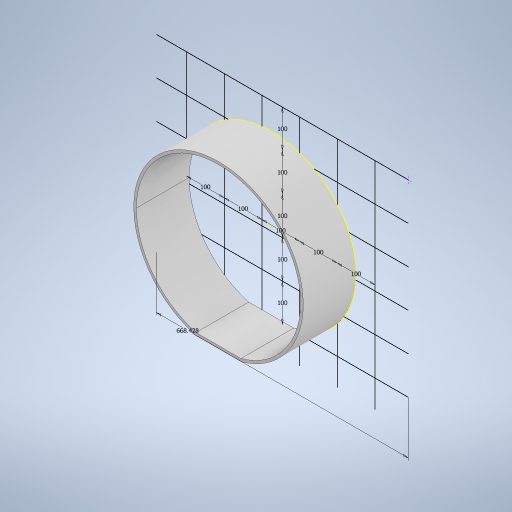
# Autodesk Inventor part: 본체
Saved by Autodesk Inventor 2023 (Build 270158000, 158)
## iProperties
Created: 2022-10-18
Part Number: 본체
Material: 일반
Document SubType Name: Sheet Metal
Designer: ghkdr
Density: 1 g/cm^3
Sheet Metal Rule: 기본값_mm
Appearance: 기본값
Author: ghkdr
Autodesk Inventor part; units mm, degrees
ref_plane "YZ Plane" through (0, 0, 0) normal (1, 0, 0) x (0, 1, 0)
ref_plane "XZ Plane" through (0, 0, 0) normal (0, 1, 0) x (-1, 0, 0)
ref_plane "XY Plane" through (0, 0, 0) normal (0, 0, 1) x (1, 0, 0)
sketch "스케치1" plane through (0, 0, 0) normal (0, 0, 1) x (1, 0, 0)
  line L0 (0.6532, 285.5724) -> (608.6579, 285.5724)
  circle A0 centre (304.6555, 285.5724) radius 26
  spline S0 degree 3 poles (86.6555, 285.5724) (86.6555, 279.2201) (86.9408, 272.7726) (88.3516, 257.3036) (89.7551, 248.2286) (93.8149, 230.0774) (96.4717, 221.0019) (103.0602, 203.1009) (106.9922, 194.2762) (116.0838, 177.1357) (121.2434, 168.8206) (132.6721, 152.9416) (138.9408, 145.3783) (152.4073, 131.206) (159.6045, 124.5975) (174.7019, 112.4806) (182.6013, 106.9724) (198.8544, 97.1353) (207.2073, 92.8062) (224.1185, 85.3392) (232.6761, 82.2009) (242.4395, 79.2689) (243.6563, 78.9149) (244.8727, 78.5724) (284.3294, 78.5724) (323.7861, 78.5724) (363.6413, 78.5724) (364.0398, 78.5724) (364.4384, 78.5724) (370.5905, 80.3047) (376.756, 82.3303) (391.4225, 87.8987) (399.8982, 91.7264) (416.5023, 100.5755) (424.6301, 105.597) (440.2863, 116.7839) (447.814, 122.9492) (462.031, 136.3053) (468.7195, 143.4958) (481.0552, 158.7216) (486.7018, 166.7563) (496.8069, 183.4416) (501.2652, 192.0915) (508.9155, 209.752) (512.1076, 218.7618) (517.2191, 236.884) (519.1388, 245.9959) (521.7638, 264.0837) (522.4696, 273.0593) (522.6361, 282.6064) (522.6452, 283.3458) (522.6528, 284.4297) (522.6543, 284.7752) (522.6554, 285.278) (522.6556, 285.4441) (522.6555, 285.7395) (522.6554, 285.8872) (522.6543, 286.3307) (522.653, 286.6267) (522.647, 287.5152) (522.6404, 288.1086) (522.6125, 289.8917) (522.5833, 291.0845) (522.463, 294.6739) (522.3394, 297.0818) (521.8333, 304.3448) (521.3155, 309.2392) (519.371, 322.7347) (517.5545, 331.408) (512.6658, 348.7558) (509.593, 357.4298) (502.1569, 374.5328) (497.7932, 382.9611) (487.8114, 399.3127) (482.1931, 407.2352) (469.8134, 422.3247) (463.0523, 429.491) (448.5685, 442.8526) (440.8466, 449.0474) (424.6771, 460.3064) (416.2304, 465.3703) (398.8783, 474.2776) (389.9738, 478.1209) (371.9775, 484.5696) (362.8865, 487.1752) (344.7692, 491.1969) (335.7435, 492.6135) (323.7617, 493.7895) (320.6828, 494.0275) (315.1548, 494.3434) (312.6985, 494.4433) (308.7237, 494.5412) (307.196, 494.5633) (304.5189, 494.5753) (303.3662, 494.5717) (301.0484, 494.5468) (299.8859, 494.5254) (296.388, 494.4341) (294.0421, 494.3369) (286.9678, 493.9326) (282.2025, 493.5126) (268.4474, 491.8509) (259.3706, 490.211) (241.1969, 485.7233) (232.1004, 482.8751) (214.146, 475.9332) (205.2888, 471.8394) (188.0871, 462.4373) (179.7435, 457.1292) (163.8338, 445.4029) (156.2685, 438.9851) (142.1441, 425.2124) (135.5858, 417.8581) (123.6456, 402.4379) (118.264, 394.3729) (108.7751, 377.7874) (104.6676, 369.2678) (97.748, 352.0342) (94.9356, 343.3209) (90.5582, 325.9429) (88.9926, 317.2786) (87.0856, 300.8895) (86.6555, 293.1449) (86.6555, 285.5724) knots 0 0 0 0 0.095101 0.095101 0.226105 0.226105 0.357108 0.357108 0.488112 0.488112 0.619116 0.619116 0.75012 0.75012 0.881123 0.881123 1.012127 1.012127 1.143131 1.143131 1.274135 1.274135 1.292791 1.292791 1.292791 2.267161 2.267161 2.277003 2.277003 2.277003 2.371364 2.371364 2.502473 2.502473 2.633583 2.633583 2.764692 2.764692 2.895802 2.895802 3.026911 3.026911 3.158021 3.158021 3.28913 3.28913 3.42024 3.42024 3.551349 3.551349 3.562375 3.562375 3.567539 3.567539 3.569898 3.569898 3.572256 3.572256 3.576972 3.576972 3.586405 3.586405 3.60527 3.60527 3.643 3.643 3.71846 3.71846 3.84958 3.84958 3.980701 3.980701 4.111821 4.111821 4.242942 4.242942 4.374062 4.374062 4.505183 4.505183 4.636303 4.636303 4.767424 4.767424 4.898544 4.898544 5.029664 5.029664 5.075343 5.075343 5.112232 5.112232 5.13541 5.13541 5.153021 5.153021 5.170631 5.170631 5.205852 5.205852 5.276293 5.276293 5.407713 5.407713 5.539132 5.539132 5.670552 5.670552 5.801971 5.801971 5.933391 5.933391 6.06481 6.06481 6.19623 6.19623 6.327649 6.327649 6.459069 6.459069 6.590488 6.590488 6.711387 6.711387 6.711387 6.711387
  line L1 (86.6555, 285.5724) -> (86.6555, 279.2201) construction
  line L2 (86.6555, 279.2201) -> (86.9408, 272.7726) construction
  line L3 (86.9408, 272.7726) -> (88.3516, 257.3036) construction
  line L4 (88.3516, 257.3036) -> (89.7551, 248.2286) construction
  line L5 (89.7551, 248.2286) -> (93.8149, 230.0774) construction
  line L6 (93.8149, 230.0774) -> (96.4717, 221.0019) construction
  line L7 (96.4717, 221.0019) -> (103.0602, 203.1009) construction
  line L8 (103.0602, 203.1009) -> (106.9922, 194.2762) construction
  line L9 (106.9922, 194.2762) -> (116.0838, 177.1357) construction
  line L10 (116.0838, 177.1357) -> (121.2434, 168.8206) construction
  line L11 (121.2434, 168.8206) -> (132.6721, 152.9416) construction
  line L12 (132.6721, 152.9416) -> (138.9408, 145.3783) construction
  line L13 (138.9408, 145.3783) -> (152.4073, 131.206) construction
  line L14 (152.4073, 131.206) -> (159.6045, 124.5975) construction
  line L15 (159.6045, 124.5975) -> (174.7019, 112.4806) construction
  line L16 (174.7019, 112.4806) -> (182.6013, 106.9724) construction
  line L17 (182.6013, 106.9724) -> (198.8544, 97.1353) construction
  line L18 (198.8544, 97.1353) -> (207.2073, 92.8062) construction
  line L19 (207.2073, 92.8062) -> (224.1185, 85.3392) construction
  line L20 (224.1185, 85.3392) -> (232.6761, 82.2009) construction
  line L21 (232.6761, 82.2009) -> (242.4395, 79.2689) construction
  line L22 (242.4395, 79.2689) -> (243.6563, 78.9149) construction
  line L23 (243.6563, 78.9149) -> (244.8727, 78.5724) construction
  line L24 (244.8727, 78.5724) -> (284.3294, 78.5724) construction
  line L25 (284.3294, 78.5724) -> (323.7861, 78.5724) construction
  line L26 (323.7861, 78.5724) -> (363.6413, 78.5724) construction
  line L27 (363.6413, 78.5724) -> (364.0398, 78.5724) construction
  line L28 (364.0398, 78.5724) -> (364.4384, 78.5724) construction
  line L29 (364.4384, 78.5724) -> (370.5905, 80.3047) construction
  line L30 (370.5905, 80.3047) -> (376.756, 82.3303) construction
  line L31 (376.756, 82.3303) -> (391.4225, 87.8987) construction
  line L32 (391.4225, 87.8987) -> (399.8982, 91.7264) construction
  line L33 (399.8982, 91.7264) -> (416.5023, 100.5755) construction
  line L34 (416.5023, 100.5755) -> (424.6301, 105.597) construction
  line L35 (424.6301, 105.597) -> (440.2863, 116.7839) construction
  line L36 (440.2863, 116.7839) -> (447.814, 122.9492) construction
  line L37 (447.814, 122.9492) -> (462.031, 136.3053) construction
  line L38 (462.031, 136.3053) -> (468.7195, 143.4958) construction
  line L39 (468.7195, 143.4958) -> (481.0552, 158.7216) construction
  line L40 (481.0552, 158.7216) -> (486.7018, 166.7563) construction
  line L41 (486.7018, 166.7563) -> (496.8069, 183.4416) construction
  line L42 (496.8069, 183.4416) -> (501.2652, 192.0915) construction
  line L43 (501.2652, 192.0915) -> (508.9155, 209.752) construction
  line L44 (508.9155, 209.752) -> (512.1076, 218.7618) construction
  line L45 (512.1076, 218.7618) -> (517.2191, 236.884) construction
  line L46 (517.2191, 236.884) -> (519.1388, 245.9959) construction
  line L47 (519.1388, 245.9959) -> (521.7638, 264.0837) construction
  line L48 (521.7638, 264.0837) -> (522.4696, 273.0593) construction
  line L49 (522.4696, 273.0593) -> (522.6361, 282.6064) construction
  line L50 (522.6361, 282.6064) -> (522.6452, 283.3458) construction
  line L51 (522.6452, 283.3458) -> (522.6528, 284.4297) construction
  line L52 (522.6528, 284.4297) -> (522.6543, 284.7752) construction
  line L53 (522.6543, 284.7752) -> (522.6554, 285.278) construction
  line L54 (522.6554, 285.278) -> (522.6556, 285.4441) construction
  line L55 (522.6556, 285.4441) -> (522.6555, 285.7395) construction
  line L56 (522.6555, 285.7395) -> (522.6554, 285.8872) construction
  line L57 (522.6554, 285.8872) -> (522.6543, 286.3307) construction
  line L58 (522.6543, 286.3307) -> (522.653, 286.6267) construction
  line L59 (522.653, 286.6267) -> (522.647, 287.5152) construction
  line L60 (522.647, 287.5152) -> (522.6404, 288.1086) construction
  line L61 (522.6404, 288.1086) -> (522.6125, 289.8917) construction
  line L62 (522.6125, 289.8917) -> (522.5833, 291.0845) construction
  line L63 (522.5833, 291.0845) -> (522.463, 294.6739) construction
  line L64 (522.463, 294.6739) -> (522.3394, 297.0818) construction
  line L65 (522.3394, 297.0818) -> (521.8333, 304.3448) construction
  line L66 (521.8333, 304.3448) -> (521.3155, 309.2392) construction
  line L67 (521.3155, 309.2392) -> (519.371, 322.7347) construction
  line L68 (519.371, 322.7347) -> (517.5545, 331.408) construction
  line L69 (517.5545, 331.408) -> (512.6658, 348.7558) construction
  line L70 (512.6658, 348.7558) -> (509.593, 357.4298) construction
  line L71 (509.593, 357.4298) -> (502.1569, 374.5328) construction
  line L72 (502.1569, 374.5328) -> (497.7932, 382.9611) construction
  line L73 (497.7932, 382.9611) -> (487.8114, 399.3127) construction
  line L74 (487.8114, 399.3127) -> (482.1931, 407.2352) construction
  line L75 (482.1931, 407.2352) -> (469.8134, 422.3247) construction
  line L76 (469.8134, 422.3247) -> (463.0523, 429.491) construction
  line L77 (463.0523, 429.491) -> (448.5685, 442.8526) construction
  line L78 (448.5685, 442.8526) -> (440.8466, 449.0474) construction
  line L79 (440.8466, 449.0474) -> (424.6771, 460.3064) construction
  line L80 (424.6771, 460.3064) -> (416.2304, 465.3703) construction
  line L81 (416.2304, 465.3703) -> (398.8783, 474.2776) construction
  line L82 (398.8783, 474.2776) -> (389.9738, 478.1209) construction
  line L83 (389.9738, 478.1209) -> (371.9775, 484.5696) construction
  line L84 (371.9775, 484.5696) -> (362.8865, 487.1752) construction
  line L85 (362.8865, 487.1752) -> (344.7692, 491.1969) construction
  line L86 (344.7692, 491.1969) -> (335.7435, 492.6135) construction
  line L87 (335.7435, 492.6135) -> (323.7617, 493.7895) construction
  line L88 (323.7617, 493.7895) -> (320.6828, 494.0275) construction
  line L89 (320.6828, 494.0275) -> (315.1548, 494.3434) construction
  line L90 (315.1548, 494.3434) -> (312.6985, 494.4433) construction
  line L91 (312.6985, 494.4433) -> (308.7237, 494.5412) construction
  line L92 (308.7237, 494.5412) -> (307.196, 494.5633) construction
  line L93 (307.196, 494.5633) -> (304.5189, 494.5753) construction
  line L94 (304.5189, 494.5753) -> (303.3662, 494.5717) construction
  line L95 (303.3662, 494.5717) -> (301.0484, 494.5468) construction
  line L96 (301.0484, 494.5468) -> (299.8859, 494.5254) construction
  line L97 (299.8859, 494.5254) -> (296.388, 494.4341) construction
  line L98 (296.388, 494.4341) -> (294.0421, 494.3369) construction
  line L99 (294.0421, 494.3369) -> (286.9678, 493.9326) construction
  line L100 (286.9678, 493.9326) -> (282.2025, 493.5126) construction
  line L101 (282.2025, 493.5126) -> (268.4474, 491.8509) construction
  line L102 (268.4474, 491.8509) -> (259.3706, 490.211) construction
  line L103 (259.3706, 490.211) -> (241.1969, 485.7233) construction
  line L104 (241.1969, 485.7233) -> (232.1004, 482.8751) construction
  line L105 (232.1004, 482.8751) -> (214.146, 475.9332) construction
  line L106 (214.146, 475.9332) -> (205.2888, 471.8394) construction
  line L107 (205.2888, 471.8394) -> (188.0871, 462.4373) construction
  line L108 (188.0871, 462.4373) -> (179.7435, 457.1292) construction
  line L109 (179.7435, 457.1292) -> (163.8338, 445.4029) construction
  line L110 (163.8338, 445.4029) -> (156.2685, 438.9851) construction
  line L111 (156.2685, 438.9851) -> (142.1441, 425.2124) construction
  line L112 (142.1441, 425.2124) -> (135.5858, 417.8581) construction
  line L113 (135.5858, 417.8581) -> (123.6456, 402.4379) construction
  line L114 (123.6456, 402.4379) -> (118.264, 394.3729) construction
  line L115 (118.264, 394.3729) -> (108.7751, 377.7874) construction
  line L116 (108.7751, 377.7874) -> (104.6676, 369.2678) construction
  line L117 (104.6676, 369.2678) -> (97.748, 352.0342) construction
  line L118 (97.748, 352.0342) -> (94.9356, 343.3209) construction
  line L119 (94.9356, 343.3209) -> (90.5582, 325.9429) construction
  line L120 (90.5582, 325.9429) -> (88.9926, 317.2786) construction
  line L121 (88.9926, 317.2786) -> (87.0856, 300.8895) construction
  line L122 (87.0856, 300.8895) -> (86.6555, 293.1449) construction
  line L123 (86.6555, 293.1449) -> (86.6555, 285.5724) construction
  spline S1 degree 2 poles (79.6555, 285.5724) (79.6555, 117.0637) (243.9137, 71.5724) (304.6555, 71.5724) (365.3974, 71.5724) (529.6555, 117.0637) (529.6555, 285.5724) (529.6555, 501.5724) (304.6555, 501.5724) (79.6555, 501.5724) (79.6555, 285.5724) knots 0 0 0 1.297441 1.297441 2.297441 2.297441 3.594882 3.594882 5.165678 5.165678 6.736475 6.736475 6.736475 weights 1 0.796857 1 1 1 0.796857 1 0.707107 1 0.707107 1
  line L124 (79.6555, 285.5724) -> (79.6555, 117.0637) construction
  line L125 (79.6555, 117.0637) -> (243.9137, 71.5724) construction
  line L126 (243.9137, 71.5724) -> (304.6555, 71.5724) construction
  line L127 (304.6555, 71.5724) -> (365.3974, 71.5724) construction
  line L128 (365.3974, 71.5724) -> (529.6555, 117.0637) construction
  line L129 (529.6555, 117.0637) -> (529.6555, 285.5724) construction
  line L130 (529.6555, 285.5724) -> (529.6555, 501.5724) construction
  line L131 (529.6555, 501.5724) -> (304.6555, 501.5724) construction
  line L132 (304.6555, 501.5724) -> (79.6555, 501.5724) construction
  line L133 (79.6555, 501.5724) -> (79.6555, 285.5724) construction
  line L134 (246.6555, 209.5724) -> (362.6555, 209.5724)
  line L135 (246.6555, 189.5724) -> (362.6555, 189.5724)
  line L136 (246.6555, 209.5724) -> (246.6555, 189.5724)
  line L137 (362.6555, 209.5724) -> (362.6555, 189.5724)
  point P0 (0, 0)
  dimension "d1" = 225
  dimension "d3" = 52
  dimension "d5" = 20
  constraints: 10 end point, 2 point on line, 1 centre point, 3 other
  measures "d1" distance of A0.centre L124.start
  measures "d3" diameter of A0
  measures "d5" distance of L134.end L135.end
extrude "돌출1" add sketch "스케치1" along normal blind 140 contours S1 L0 S0 | L0 S0 S1
sketch "스케치2" plane through (0, 0, 0) normal (0, 0, -1) x (-1, 0, 0)
  ellipse E0 centre (-304.6555, 285.5724) end of major axis (-529.6555, 285.5724) minor radius 222.2521 (-243.9137, 71.5724) -> (-79.6555, 285.5724) ccw projected
  line L0 (-243.9137, 71.5724) -> (-365.3974, 71.5724) projected
  line L1 (-179.6555, 0) -> (-179.6555, 571.5724)
  line L2 (-279.6555, 0) -> (-279.6555, 571.5724)
  line L3 (-379.6555, 0) -> (-379.6555, 571.5724)
  line L4 (-479.6555, 0) -> (-479.6555, 571.5724)
  line L5 (-579.6555, 0) -> (-579.6555, 571.5724)
  line L6 (0, 71.5724) -> (-668.4284, 71.5724)
  line L7 (0, 171.5724) -> (-668.4284, 171.5724)
  line L8 (0, 271.5724) -> (-668.4284, 271.5724)
  line L9 (0, 371.5724) -> (-668.4284, 371.5724)
  line L10 (0, 471.5724) -> (-668.4284, 471.5724)
  line L11 (0, 571.5724) -> (-668.4284, 571.5724)
  line L12 (-79.6555, 0) -> (-79.6555, 571.5724)
  point P0 (0, 0)
  dimension "d10" = 100
  dimension "d11" = 100
  dimension "d12" = 100
  dimension "d13" = 100
  dimension "d15" = 100
  dimension "d16" = 100
  dimension "d17" = 100
  dimension "d18" = 100
  dimension "d19" = 100
  dimension "d20" = 100
  dimension "d21" = 668.4284
  constraints: 24 end point, 10 parallel, 6 point on line, 1 vertical, 5 other
  measures "d10" distance between parallel lines of L1 L2
  measures "d11" distance between parallel lines of L2 L3
  measures "d12" distance between parallel lines of L3 L4
  measures "d13" distance between parallel lines of L4 L5
  measures "d15" distance between parallel lines of L6 L7
  measures "d16" distance between parallel lines of L7 L8
  measures "d17" distance between parallel lines of L8 L9
  measures "d18" distance between parallel lines of L9 L10
  measures "d19" distance between parallel lines of L10 L11
  measures "d20" distance between parallel lines of L1 L12
  measures "d21" distance of L6.start L6.end
equation "\"TransitionRadius\" = BendRadius"
equation "\"BendRadius\" = 0.5"
